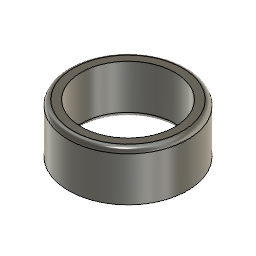
SunSpacer (Autodesk Fusion 360 design; units mm, degrees)
Autodesk Fusion 360 part; units mm, degrees
sketch "Sketch1" plane through (0, 0, 0) normal (0, 0, 1) x (1, 0, 0)
  circle A0 centre (0, 0) radius 4.775
  circle A1 centre (0, 0) radius 6.05
  dimension "d5" = 9.55
  dimension "d6" = 12.1
  constraint coincident A0.centre A1.centre
  constraint concentric A0 A1
  measures "d5" diameter of A0
  measures "d6" diameter of A1
extrude "Extrude1" add sketch "Sketch1" along normal blind 5
fillet "Fillet1" radius 0.5 2 edges at (-5.6406, -2.1878, 5) (-4.4519, 1.7267, 0)
equation "bearing_id = 12 mm"
equation "sun_shaft_od = 9.5 mm"
equation "sun_shaft_clearance = 0.05 mm"
equation "bearing_id_clearance = 0.1 mm"
equation "d5 = sun_shaft_od + sun_shaft_clearance"
equation "d6 = bearing_id + bearing_id_clearance"
equation "height = 5 mm"
equation "d8 = height"
